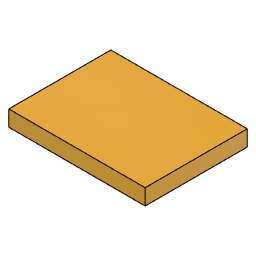
Naustok (Autodesk Fusion 360 archive; units mm, degrees)
design "GY-68"
Autodesk Fusion 360 part; units mm, degrees
sketch "Sketch1" plane through (0, 0, 0) normal (0, 1, 0) x (1, 0, 0)
  line L0 (7.75, 5.8) -> (-7.75, 5.8)
  line L1 (-7.75, 5.8) -> (-7.75, -5.8)
  line L2 (-7.75, -5.8) -> (7.75, -5.8)
  line L3 (7.75, -5.8) -> (7.75, 5.8)
  line L4 (7.75, 5.8) -> (-7.75, -5.8) construction
  line L5 (-7.75, 5.8) -> (7.75, -5.8) construction
  dimension "d1" = 15.5
  dimension "d2" = 11.6
  constraint horizontal L0
  constraint perpendicular L0 L1
  constraint parallel L0 L2
  constraint parallel L1 L3
  constraint coincident L4 origin
  constraint coincident L5 origin
  measures "d1" distance of L1 L3
  measures "d2" distance of L0 L2
extrude "Extrude1" add sketch "Sketch1" along normal blind 1.8
